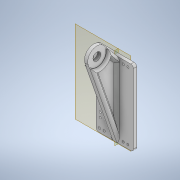
# Autodesk Inventor part: Fastener
Saved by Autodesk Inventor 2022 (Build 260153000, 153)
## iProperties
Created: 2023-10-19
Part Number: Fastener
Material: Типовые
Document SubType Name: Modeling
Designer: user
Density: 1 g/cm^3
Appearance: По умолчанию
Author: user
## iProperties of the stored document Fastener horizontal_3DПЕЧАТЬ.ipt
Created: 2023-10-22
Part Number: Fastener horizontal_3DПЕЧАТЬ
Material: Типовые
Document SubType Name: Modeling
Designer: user
Density: 1 g/cm^3
Appearance: По умолчанию
Author: user
Autodesk Inventor part; units mm, degrees
ref_plane "YZ Plane" through (0, 0, 0) normal (1, 0, 0) x (0, 1, 0)
ref_plane "XZ Plane" through (0, 0, 0) normal (0, 1, 0) x (-1, 0, 0)
ref_plane "XY Plane" through (0, 0, 0) normal (0, 0, 1) x (1, 0, 0)
ref_plane "РабПлоскость1" through (0, 0, 0) normal (0, 0, 1) x (1, 0, 0)
sketch "Эскиз1" plane through (0, 0, 0) normal (0, 0, 1) x (1, 0, 0)
  line L0 (15.9535, 22.685) -> (15.9535, 17.285) projected
  line L1 (15.9535, 17.285) -> (5.5535, 17.285) projected
  line L2 (5.5535, 17.285) -> (5.5535, 22.685) projected
  line L3 (5.5535, 22.685) -> (15.9535, 22.685) projected
  line L4 (15.9535, -17.315) -> (15.9535, -22.715) projected
  line L5 (15.9535, -22.715) -> (5.5535, -22.715) projected
  line L6 (5.5535, -22.715) -> (5.5535, -17.315) projected
  line L7 (5.5535, -17.315) -> (15.9535, -17.315) projected
  arc A0 (-2.3465, 28.685) -> (-4.3465, 26.685) centre (-2.3465, 26.685) ccw projected
  line L8 (-4.3465, 12.1) -> (-4.3465, 26.685) projected
  arc A1 (-5.6809, 10.2141) -> (-4.3465, 12.1) centre (-6.3465, 12.1) ccw projected
  line L9 (-11.5122, 8.156) -> (-5.6809, 10.2141) projected
  arc A2 (-11.5122, 8.156) -> (-12.8465, 6.27) centre (-10.8465, 6.27) ccw projected
  line L10 (-12.8465, -1.915) -> (-12.8465, 6.27) projected
  arc A3 (-12.8465, -1.915) -> (-10.8465, -3.915) centre (-10.8465, -1.915) ccw projected
  line L11 (-4.6465, -3.915) -> (-10.8465, -3.915) projected
  arc A4 (-2.6465, -5.915) -> (-4.6465, -3.915) centre (-4.6465, -5.915) ccw projected
  line L12 (-2.6465, -26.715) -> (-2.6465, -5.915) projected
  arc A5 (-2.6465, -26.715) -> (-0.6465, -28.715) centre (-0.6465, -26.715) ccw projected
  line L13 (23.8535, -28.715) -> (-0.6465, -28.715) projected
  arc A6 (23.8535, -28.715) -> (25.8535, -26.715) centre (23.8535, -26.715) ccw projected
  line L14 (25.8535, 26.685) -> (25.8535, -26.715) projected
  arc A7 (25.8535, 26.685) -> (23.8535, 28.685) centre (23.8535, 26.685) ccw projected
  line L15 (-2.3465, 28.685) -> (23.8535, 28.685) projected
  circle A8 centre (18.0535, 25.685) radius 0.8 projected
  circle A9 centre (21.6535, 25.685) radius 0.8 projected
  circle A10 centre (21.6535, -25.715) radius 0.8 projected
  circle A11 centre (18.0535, -25.715) radius 0.8 projected
  circle A12 centre (0.3535, -18.515) radius 0.8 projected
  circle A13 centre (0.3535, -14.915) radius 0.8 projected
  circle A14 centre (-1.3465, 16.885) radius 0.8 projected
  circle A15 centre (-1.3465, 20.485) radius 0.8 projected
  circle A16 centre (-0.1465, 25.685) radius 0.8 projected
  circle A17 centre (3.4535, 25.685) radius 0.8 projected
  circle A18 centre (-0.1465, -25.715) radius 0.8 projected
  circle A19 centre (3.4535, -25.715) radius 0.8 projected
  line L16 (-4.3465, 12.1) -> (-2.6465, -5.915)
  circle A20 centre (51.6035, 35.685) radius 3
  circle A21 centre (51.6035, 35.685) radius 6
  line L17 (11.6035, -28.715) -> (11.6035, 28.685) construction
  line L18 (56.9244, 32.9123) -> (25.8535, -26.715)
  line L19 (50.1799, 41.5137) -> (-2.3465, 28.685)
  point P0 (0, 0)
  point P1 (-2.6818, -5.5409)
  dimension "d11" = 6
  dimension "d12" = 12
  dimension "d13" = 7
  dimension "d14" = 40
  constraints: 8 end point, 2 centre point, 2 point on circle, 2 tangent, 1 coincident, 1 midpoint, 1 perpendicular, 1 point on line
  measures "d11" diameter of A20
  measures "d12" diameter of A21
  measures "d13" distance from line of L15 A20.centre
  measures "d14" distance from line of A20.centre L17
extrude "Выдавливание1" add sketch "Эскиз1" along normal blind 2.5 contours L0 L1 L2 L3 | L4 L5 L6 L7 | L15 A7 L14 A6 L13 A5 L12 A4 L16 L8 A0
ref_plane "РабПлоскость3" through (11.6035, -26.715, 0) normal (-1, 0, 0) x (0, 0, 1)
sketch "Эскиз6" plane through (11.6035, -26.715, 0) normal (-1, 0, 0) x (0, 0, 1)
  circle A0 centre (17.5, 62.4) radius 3
  circle A1 centre (17.5, 62.4) radius 7
  line L0 (0, 55.4) -> (2.5, 55.4) projected
  line L1 (12.135, 66.8964) -> (2.5, 55.4)
  line L2 (24.1111, 60.0993) -> (2.5, -2)
  line L3 (2.5, 0) -> (2.5, 53.4) projected
  line L4 (2.5, -2) -> (2.5, 0) projected
  line L5 (2.5, 53.4) -> (2.5, 55.4) projected
  line L6 (2.5, 4.085) -> (19.7626, 53.6891)
  line L7 (8.8611, 59.8763) -> (2.5, 52.2864)
  line L8 (2.5, 20.8) -> (2.5, 0) projected
  line L9 (2.5, 53.4) -> (2.5, 38.815) projected
  arc A2 (8.8611, 59.8763) -> (19.7626, 53.6891) centre (17.5, 62.4) ccw
  line L10 (23.1251, 57.2659) -> (10.208, 64.5971)
  point P0 (0, 26.715)
  point P1 (2.5, 52.2864)
  point P2 (22.5746, 57.5784)
  point P3 (10.7585, 64.2847)
  dimension "d30" = 6
  dimension "d31" = 14
  dimension "d32" = 7
  dimension "d33" = 15
  dimension "d34" = 2
  dimension "d35" = 2
  dimension "d36" = 2
  dimension "d46" = 3
  dimension "d47" = 3
  constraints: 10 end point, 4 point on circle, 4 point on line, 3 centre point, 2 coincident, 2 parallel, 2 tangent
  measures "d30" diameter of A0
  measures "d31" diameter of A1
  measures "d32" distance from line of A0.centre L0
  measures "d33" distance from line of A0.centre L3
  measures "d34" distance between parallel lines of L2 L6
  measures "d35" distance between parallel lines of L1 L7
  measures "d36" radial gap between concentric circles of A1 A2
  measures "d46" distance of L2.start L10.start
  measures "d47" distance of L10.end L1.start
extrude "Выдавливание3" add sketch "Эскиз6" along normal mid plane 2.5 contours A0 L10 A1 | A0 L10 A1 | L10 L1 A1 | A1 L10 L2 L4 L3 L6 A2 L7 L5 L1 | A1 L2 L10 | L7 A2 L6 L3
extrude "Выдавливание4" add sketch "Эскиз6" along normal mid plane 7 contours A1 L10 L2 L4 L3 L6 A2 L7 L5 L1
fillet "Сопряжение2" radius 2 6 edges at (8.1035, 0.918, 12.8125) (15.1035, 0.918, 12.8125) (8.1035, 33.2836, 6.354) (15.1035, 33.2836, 6.354) (8.1035, 29.5972, 14.0448) (15.1035, 29.5972, 14.0448)
chamfer "Фаска1" distance 2 angle 45 6 edges at (10.3535, 2.1721, 11.1313) (12.8535, 2.1721, 11.1313) (12.8535, 1.4707, 2.5) (10.3535, 1.4707, 2.5) (10.3535, 29.3663, 5.6805) (12.8535, 29.3663, 5.6805)
